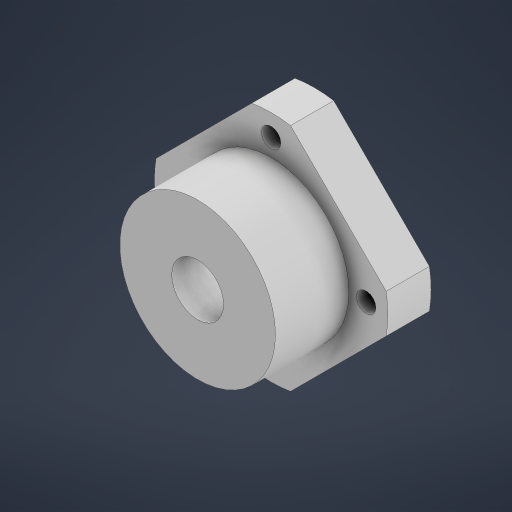
# Autodesk Inventor part: FK12
Saved by Autodesk Inventor 2023 (Build 270158000, 158)
## iProperties
Created: 2025-09-03
Part Number: FK12
Material: 일반
Document SubType Name: Modeling
Designer: k
Density: 1 g/cm^3
Appearance: 기본값
Author: k
Autodesk Inventor part; units mm, degrees
ref_plane "YZ Plane" through (0, 0, 0) normal (1, 0, 0) x (0, 1, 0)
ref_plane "XZ Plane" through (0, 0, 0) normal (0, 1, 0) x (-1, 0, 0)
ref_plane "XY Plane" through (0, 0, 0) normal (0, 0, 1) x (1, 0, 0)
sketch "스케치2" plane through (0, 0, 0) normal (0, 0, 1) x (1, 0, 0)
  circle A0 centre (-31.6118, 31.843) radius 22
  line L0 (-27.1234, 5.2186) -> (-4.9875, 27.3546)
  line L1 (-27.1234, 58.4673) -> (-4.9875, 36.3313)
  line L2 (-58.2361, 36.3313) -> (-36.1001, 58.4673)
  line L3 (-58.2361, 27.3546) -> (-36.1001, 5.2186)
  arc A1 (-27.1234, 58.4673) -> (-36.1001, 58.4673) centre (-31.6118, 31.843) ccw
  arc A2 (-58.2361, 36.3313) -> (-58.2361, 27.3546) centre (-31.6118, 31.843) ccw
  arc A3 (-36.1001, 5.2186) -> (-27.1234, 5.2186) centre (-31.6118, 31.843) ccw
  arc A4 (-4.9875, 27.3546) -> (-4.9875, 36.3313) centre (-31.6118, 31.843) ccw
  circle A5 centre (-31.6118, 53.843) radius 2.25
  circle A6 centre (-53.6118, 31.843) radius 2.25
  circle A7 centre (-31.6118, 9.843) radius 2.25
  circle A8 centre (-9.6118, 31.843) radius 2.25
  point P0 (0, 0)
  dimension "d1" = 44
  dimension "d8" = 27
  dimension "d9" = 4.5
  dimension "d10" = 4.5
  dimension "d11" = 4.5
  dimension "d12" = 4.5
  constraints: 12 point on circle, 9 centre point, 8 end point, 2 parallel, 1 coincident
  measures "d1" diameter of A0
  measures "d8" radius of A1
  measures "d9" diameter of A5
  measures "d10" diameter of A6
  measures "d11" diameter of A7
  measures "d12" diameter of A8
extrude "돌출1" add sketch "스케치2" along normal blind 10 contours A8 A0 A7 A6 A5 | A0 L1 A4 L0 A8 | A0 A5 L2 A1 L1 | L0 A3 L3 A0 A7 | A0 A6 L3 A2 L2
sketch "스케치3" plane through (0, 0, 10) normal (0, 0, 1) x (1, 0, 0)
  arc A0 (-4.9875, 27.3546) -> (-4.9875, 36.3313) centre (-31.6118, 31.843) ccw projected
  circle A1 centre (-31.6118, 31.843) radius 18
  point P0 (0, 0)
  dimension "d16" = 36
  constraints: 1 centre point, 1 coincident
  measures "d16" diameter of A1
extrude "돌출2" add sketch "스케치3" along normal blind 17
sketch "스케치4" plane through (-31.6118, 31.843, 27) normal (0, 0, 1) x (1, 0, 0)
  circle A0 centre (0, 0) radius 18 projected
  circle A1 centre (0, 0) radius 6
  point P0 (31.6118, -31.843)
  dimension "d19" = 12
  constraints: 1 centre point, 1 coincident
  measures "d19" diameter of A1
extrude "돌출3" cut sketch "스케치4" against normal through all contours A1
sketch "스케치5" plane through (0, 0, 0) normal (0, 0, -1) x (-1, 0, 0)
  circle A0 centre (53.6118, 31.843) radius 2.25 projected
  circle A1 centre (53.6118, 31.843) radius 4
  circle A2 centre (31.6118, 53.843) radius 2.25 projected
  circle A3 centre (31.6118, 53.843) radius 4
  circle A4 centre (9.6118, 31.843) radius 2.25 projected
  circle A5 centre (9.6118, 31.843) radius 4
  circle A6 centre (31.6118, 9.843) radius 2.25 projected
  circle A7 centre (31.6118, 9.843) radius 4
  point P0 (0, 0)
  dimension "d26" = 8
  dimension "d27" = 8
  dimension "d28" = 8
  dimension "d29" = 8
  constraints: 4 centre point, 4 coincident
  measures "d26" diameter of A1
  measures "d27" diameter of A3
  measures "d28" diameter of A5
  measures "d29" diameter of A7
extrude "돌출4" cut sketch "스케치5" against normal blind 4 contours A0 | A1 | A2 | A3 | A4 | A5 | A6 | A7
